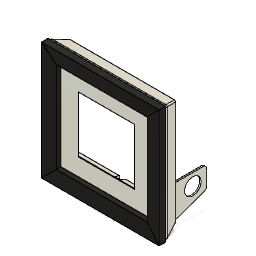
3D_Model (Autodesk Fusion 360 design; units mm, degrees)
Autodesk Fusion 360 part; units mm, degrees
note: some values were not read from the file. Set by a fixed rule: which sketch regions a step uses.
sketch "Sketch1" plane through (0, 0, 0) normal (0, 0, 1) x (1, 0, 0)
  line L0 (-57.45, 42.9) -> (57.45, 42.9)
  line L1 (57.45, 42.9) -> (57.45, -42.9)
  line L2 (57.45, -42.9) -> (-57.45, -42.9)
  line L3 (-57.45, -42.9) -> (-57.45, 42.9)
  line L4 (-57.45, 42.9) -> (57.45, -42.9) construction
  line L5 (57.45, 42.9) -> (-57.45, -42.9) construction
  line L6 (-63, 47.85) -> (63, 47.85)
  line L7 (63, 47.85) -> (63, -52.15)
  line L8 (63, -52.15) -> (-63, -52.15)
  line L9 (-63, -52.15) -> (-63, 47.85)
  line L10 (-57.45, 0) -> (-63, 0)
  line L11 (57.45, 0) -> (63, 0)
  dimension "d1" = 85.8
  dimension "d2" = 114.9
  dimension "d3" = 126
  dimension "d4" = 100
  dimension "d6" = 9.25
  constraint horizontal L0
  constraint perpendicular L0 L1
  constraint parallel L0 L2
  constraint parallel L1 L3
  constraint coincident L4 origin
  constraint coincident L5 origin
  constraint horizontal L6
  constraint vertical L7
  constraint horizontal L8
  constraint vertical L9
  constraint midpoint L3 L10.start
  constraint coincident L9 L10.end
  constraint perpendicular L9 L10
  constraint midpoint L1 L11.start
  constraint coincident L7 L11.end
  constraint perpendicular L7 L11
  constraint equal L10 L11
  measures "d1" distance of L0 L2
  measures "d2" distance of L0.start L0.end
  measures "d3" distance of L6.start L6.end
  measures "d4" distance of L6.start L8.end
  measures "d6" distance of L2 L8
sketch "Sketch2" plane through (0, 0, 0) normal (0, 0, 1) x (1, 0, 0)
  line L0 (42, 42) -> (-42, 42)
  line L1 (-42, 42) -> (-42, -42)
  line L2 (-42, -42) -> (42, -42)
  line L3 (42, -42) -> (42, 42)
  line L4 (42, 42) -> (-42, -42) construction
  line L5 (-42, 42) -> (42, -42) construction
  line L6 (67.956, 67.956) -> (-67.956, 67.956)
  line L7 (-67.956, 67.956) -> (-67.956, -67.956)
  line L8 (-67.956, -67.956) -> (67.956, -67.956)
  line L9 (67.956, -67.956) -> (67.956, 67.956)
  line L10 (67.956, 67.956) -> (-67.956, -67.956) construction
  line L11 (-67.956, 67.956) -> (67.956, -67.956) construction
  line L12 (-87.956, 87.956) -> (87.956, 87.956)
  line L13 (87.956, 87.956) -> (87.956, -87.956)
  line L14 (87.956, -87.956) -> (-87.956, -87.956)
  line L15 (-87.956, -87.956) -> (-87.956, 87.956)
  line L16 (-87.956, 87.956) -> (87.956, -87.956) construction
  line L17 (87.956, 87.956) -> (-87.956, -87.956) construction
  dimension "d7" = 84
  dimension "d8" = 135.912
  dimension "d9" = 20
  constraint horizontal L0
  constraint perpendicular L0 L1
  constraint parallel L0 L2
  constraint parallel L1 L3
  constraint coincident L4 origin
  constraint coincident L5 origin
  constraint equal L0 L1
  constraint horizontal L6
  constraint perpendicular L6 L7
  constraint parallel L6 L8
  constraint parallel L7 L9
  constraint coincident L10 origin
  constraint coincident L11 origin
  constraint equal L6 L9
  constraint horizontal L12
  constraint perpendicular L12 L13
  constraint parallel L12 L14
  constraint parallel L13 L15
  constraint coincident L16 origin
  constraint coincident L17 origin
  constraint equal L12 L15
  measures "d7" distance of L0.start L0.end
  measures "d8" distance of L6.end L7.end
  measures "d9" distance of L7 L15
extrude "Extrude1" add sketch "Sketch2" along normal blind 1 contours L6 L7 L8 L9 makes body 1
extrude "Extrude2" add sketch "Sketch2" along normal blind 10 separate body contours L12 L13 L14 L15 makes body 2
chamfer "Chamfer1" distance 20 distance2 2 4 edges at (0, 67.956, 10) (67.956, 0, 10) (0, -67.956, 10) (-67.956, 0, 10) measured on face at (-22.652, 81.2893, 10) measured on face at (-22.652, 81.2893, 10) measured on face at (-22.652, 81.2893, 10) measured on face at (-22.652, 81.2893, 10) on bodies 2
sketch "Sketch3" plane through (0, 0, 0) normal (0, 0, -1) x (1, 0, 0)
  line L0 (87.956, 87.956) -> (-87.956, 87.956)
  line L1 (-87.956, 87.956) -> (-87.956, -87.956)
  line L2 (-87.956, -87.956) -> (87.956, -87.956)
  line L3 (87.956, -87.956) -> (87.956, 87.956)
  line L4 (42, 42) -> (42, -42)
  line L5 (42, -42) -> (-42, -42)
  line L6 (-42, -42) -> (-42, 42)
  line L7 (-42, 42) -> (42, 42)
  line L8 (-63, 52.15) -> (-63, -47.85)
  line L9 (63, 52.15) -> (-63, 52.15)
  line L10 (-63, -47.85) -> (63, -47.85)
  line L11 (63, -47.85) -> (63, 52.15)
  line L12 (63.3, 52.45) -> (-63.3, 52.45)
  line L13 (-63.3, 52.45) -> (-63.3, -48.15)
  line L14 (-63.3, -48.15) -> (63.3, -48.15)
  line L15 (63.3, -48.15) -> (63.3, 52.45)
  line L16 (86.956, -86.956) -> (86.956, 86.956)
  line L17 (86.956, 86.956) -> (-86.956, 86.956)
  line L18 (-86.956, 86.956) -> (-86.956, -86.956)
  line L19 (-86.956, -86.956) -> (86.956, -86.956)
  line L20 (67.956, -67.956) -> (67.956, 67.956)
  line L21 (-67.956, -67.956) -> (67.956, -67.956)
  line L22 (-67.956, 67.956) -> (-67.956, -67.956)
  line L23 (67.956, 67.956) -> (-67.956, 67.956)
  line L24 (67.956, 67.956) -> (67.956, -67.956)
  line L25 (67.956, -67.956) -> (-67.956, -67.956)
  line L26 (-67.956, -67.956) -> (-67.956, 67.956)
  line L27 (-67.956, 67.956) -> (67.956, 67.956)
  dimension "d14" = 0.3
  dimension "d26" = -1
extrude "Extrude3" add sketch "Sketch3" along normal blind 3 separate body contours L16 L17 L18 L19 | L20 L21 L22 L23 L24 L25 L26 L27 makes body 3
extrude "Extrude4" add 1 faces at (-21.1, 74.0207, -3) along direction (0, 0, -1) blind 20 draft -20 on bodies 3 bodies 3
sketch "Sketch7" plane through (0, 0, 0) normal (0, 0, 1) x (1, 0, 0)
  line L0 (-63, -52.15) -> (-63, 47.85) construction
  circle A0 centre (-63, 33.35) radius 7.5
  circle A1 centre (-63, -31.65) radius 7.5
  circle A2 centre (-63, 11.35) radius 7.5
  circle A3 centre (-63, -10.15) radius 7.5
  dimension "d41" = 14.5
  dimension "d42" = 36.5
  dimension "d43" = 58
  dimension "d44" = 79.5
  dimension "d45" = 15
  constraint equal A0 A2
  constraint equal A2 A3
  constraint equal A1 A3
  constraint coincident L0 A0.centre
  constraint coincident L0 A2.centre
  constraint coincident L0 A3.centre
  constraint coincident L0 A1.centre
  measures "d41" distance of L0.end A0.centre
  measures "d42" distance of L0.end A2.centre
  measures "d43" distance of L0.end A3.centre
  measures "d44" distance of L0.end A1.centre
  measures "d45" diameter of A1
extrude "Extrude8" cut sketch "Sketch7" against normal blind 60 from surface at -3 bodies 3
sketch "Sketch5" plane through (0, 0, -23) normal (0, 0, -1) x (1, 0, 0)
  line L0 (70.5794, -55.4294) -> (-70.5794, -55.4294)
  line L1 (-70.5794, -55.4294) -> (-70.5794, 59.7294)
  line L2 (-70.5794, 59.7294) -> (70.5794, 59.7294)
  line L3 (70.5794, 59.7294) -> (70.5794, -55.4294)
  line L4 (-79.6766, 79.6766) -> (-79.6766, -79.6766)
  line L5 (-79.6766, -79.6766) -> (79.6766, -79.6766)
  line L6 (79.6766, -79.6766) -> (79.6766, 79.6766)
  line L7 (79.6766, 79.6766) -> (-79.6766, 79.6766)
  line L8 (70.5794, -55.4294) -> (-70.5794, -55.4294)
  line L9 (79.6766, -79.6766) -> (-79.6766, -79.6766)
  line L10 (0, -55.4294) -> (0, -67.553) construction
  line L11 (0, -67.553) -> (0, -79.6766) construction
  line L12 (-2.5, -61.4912) -> (-2.5, -73.6148)
  arc A0 (-2.5, -73.6148) -> (2.5, -73.6148) centre (0, -73.6148) ccw
  line L13 (2.5, -73.6148) -> (2.5, -61.4912)
  arc A1 (2.5, -61.4912) -> (-2.5, -61.4912) centre (0, -61.4912) ccw
  line L14 (0, -61.4912) -> (0, -73.6148) construction
  circle A2 centre (0, -61.4912) radius 4.5
  line L15 (-4.5, -61.4912) -> (-4.5, -73.6148)
  arc A3 (-4.5, -73.6148) -> (4.5, -73.6148) centre (0, -73.6148) ccw
  line L16 (4.5, -73.6148) -> (4.5, -61.4912)
  arc A4 (4.5, -61.4912) -> (-4.5, -61.4912) centre (0, -61.4912) ccw
  line L17 (0, -61.4912) -> (0, -73.6148) construction
  point P0 (0, -67.553)
  dimension "d29" = 2.5
  dimension "d30" = 9
  constraint midpoint L0 L10.start
  constraint midpoint L5 L11.end
  constraint perpendicular L5 L11
  constraint equal L10 L11
  constraint tangent L12 A0
  constraint tangent A0 L13
  constraint parallel L12 L13
  constraint tangent L13 A1
  constraint tangent L12 A1
  constraint midpoint L11 A0.centre
  constraint parallel L11 L14
  constraint coincident P0 L10.end
  constraint midpoint L14 P0
  constraint concentric A1 A2
  constraint tangent L15 A3
  constraint tangent A3 L16
  constraint parallel L15 L16
  constraint tangent L16 A4
  constraint tangent L15 A4
  constraint coincident A0.centre L14.end
  constraint parallel L14 L17
  constraint coincident A1.centre L14.start
  constraint coincident A2 L16.end
  measures "d29" radius of A0
  measures "d30" diameter of A2
extrude "Extrude5" cut sketch "Sketch5" against normal blind 2.5 contours L12 L13 A1 A2 | L12 L13 A1 A2 A4 | L12 A0 L13 A2 bodies 3
extrude "Extrude6" cut sketch "Sketch5" against normal blind 4 from surface at -2.5 contours L12 L13 A1 A2 | L12 L13 A1 A2 A4 | L12 A0 L13 A2 | L12 A0 L13 A2 L15 A3 L16 bodies 3
sketch "Sketch6" plane through (0, 0, 0) normal (0, 0, 1) x (1, 0, 0)
  line L0 (-1.5, -102.1737) -> (1.5, -102.1737)
  line L1 (1.5, -102.1737) -> (1.5, -31.1695)
  line L2 (1.5, -31.1695) -> (-1.5, -31.1695)
  line L3 (-1.5, -31.1695) -> (-1.5, -102.1737)
  line L4 (0, 0) -> (0, -31.1695) construction
  dimension "d36" = 3
  constraint horizontal L0
  constraint vertical L1
  constraint horizontal L2
  constraint vertical L3
  constraint coincident L4.start origin
  constraint midpoint L2 L4.end
  constraint vertical L4
  measures "d36" distance of L0.start L0.end
extrude "Extrude7" cut sketch "Sketch6" against normal blind 20 draft 10 from surface at -15 bodies 3
ref_plane "WorkPlane2" through (75.128, 0, -11.5562) normal (1, 0, 0) x (0, -1, 0)
sketch "Sketch15" plane through (75.128, 0, -14.2166) normal (1, 0, 0) x (0, 1, 0)
  line L0 (79.6766, -8.7834) -> (-79.6766, -8.7834) construction
  line L1 (-86.956, 11.2166) -> (-79.6766, -8.7834)
  line L2 (-79.8362, -8.7834) -> (-61.6377, -58.7834)
  line L3 (-79.6766, -8.7834) -> (-69.6766, -8.7834)
  line L4 (-69.6766, -8.7834) -> (-76.956, 11.2166)
  line L5 (-76.956, 11.2166) -> (-36.956, 11.2166)
  line L6 (-36.956, 11.2166) -> (-29.6766, -8.7834)
  line L7 (-29.6766, -8.7834) -> (-29.6766, -58.7834)
  line L8 (-29.6766, -58.7834) -> (-61.6377, -58.7834)
  line L9 (-79.8362, -8.7834) -> (-79.6766, -8.7834)
  line L10 (-79.622, -8.9334) -> (-69.4624, -8.9334)
  line L11 (-69.4624, -8.9334) -> (-76.7418, 11.0666)
  line L12 (-76.7418, 11.0666) -> (-37.061, 11.0666)
  line L13 (-37.061, 11.0666) -> (-29.8266, -8.8098)
  line L14 (-29.8266, -8.8098) -> (-29.8266, -58.6334)
  line L15 (-29.8266, -58.6334) -> (-61.5327, -58.6334)
  line L16 (-79.622, -8.9334) -> (-61.5327, -58.6334)
  circle A0 centre (-47.7283, -38.014) radius 12.2849
  dimension "d56" = 10
  dimension "d57" = 20
  dimension "d58" = 40
  dimension "d59" = 50
  dimension "d64" = 0.15
  dimension "d65" = -0.15
  constraint coincident L0.end L1.end
  constraint coincident L0 L3.end
  constraint parallel L0 L3
  constraint parallel L3 L5
  constraint parallel L2 L6
  constraint parallel L2 L4
  constraint coincident L0 L6.end
  constraint perpendicular L0 L7
  constraint horizontal L8
  constraint coincident L2.start L3
  constraint parallel L1 L2
  measures "d56" distance of L0.end L3.end
  measures "d57" distance of L3 L5
  measures "d58" distance of L4.end L5.end
  measures "d59" vertical distance of L2.end L2.start
  measures "d64" distance of L2 L0.end
extrude "Extrude10" cut sketch "Sketch15" along normal mid plane 2.5 contours L2 L3 L4 L5 L6 L7 L8 L9 | L10 L11 L12 L13 L14 L15 L16 | A0 bodies 3
mirror "Mirror1" about plane through (0, 0, 0) normal (1, 0, 0) of "Extrude10"
extrude "Extrude11" add sketch "Sketch15" along normal mid plane 2.2 separate body contours L10 L11 L12 L13 L14 L15 L16 makes body 4
fillet "Fillet2" radius 5 6 edges at (75.128, -61.5327, -72.85) (75.128, -29.8266, -72.85) (75.128, -76.7418, -3.15) (75.128, -37.061, -3.15) (75.128, -79.622, -23.15) (75.128, -29.8266, -23.0264) on bodies 4
fillet "Fillet3" radius 2 14 edges at (83.3163, 83.3163, -13) (86.956, 86.956, -1.5) (-83.3163, 83.3163, -13) (-86.956, 86.956, -1.5) (-83.3163, -83.3163, -13) (-86.956, -86.956, -1.5) (83.3163, -83.3163, -13) (86.956, -86.956, -1.5) (2.9106, -69.703, -23) (2.2053, -58.2735, -19) (2.2053, -81.1325, -19) (-2.2053, -81.1325, -19) (-2.9106, -69.703, -23) (-2.2053, -58.2735, -19) on bodies 3
equation "d3 = 125.4 mm + 0.6 mm"
equation "d4 = 99.5 mm + 0.5 mm"
equation "d6 = 9 mm + 0.25 mm"
equation "d8 = ( 84 * 1.618 ) * 1 mm"
named bodies: "Mount", "Frame", "Body", "Stand"
